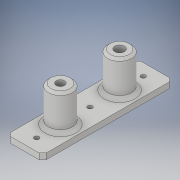
# Autodesk Inventor part: Part2
Saved by Autodesk Inventor 2019 (Build 230136000, 136)
## iProperties
Created: 2018-10-08
Part Number: Part2
Material: Generic
Document SubType Name: Modeling
Designer: Steven
Density: 1 g/cm^3
Appearance: Default
Author: Steven
## iProperties of the stored document Part2_3DPrint.ipt
Created: 2018-10-11
Part Number: Part2_3DPrint
Material: Generic
Document SubType Name: Modeling
Designer: Steven
Density: 1 g/cm^3
Appearance: Default
Author: Steven
Autodesk Inventor part; units mm, degrees
ref_plane "YZ Plane" through (0, 0, 0) normal (1, 0, 0) x (0, 1, 0)
ref_plane "XZ Plane" through (0, 0, 0) normal (0, 1, 0) x (-1, 0, 0)
ref_plane "XY Plane" through (0, 0, 0) normal (0, 0, 1) x (1, 0, 0)
sketch "Sketch1" plane through (0, 0, 0) normal (0, 1, 0) x (-1, 0, 0)
  line L0 (0, 0) -> (30, 0)
  line L1 (30, 0) -> (30, -110)
  line L2 (30, -110) -> (0, -110)
  line L3 (0, -110) -> (0, 0)
  dimension "d0" = 30
  dimension "d1" = 110
  constraints: 8 end point, 2 parallel, 1 horizontal, 1 perpendicular
  measures "d0" distance of L1.end L2.end
  measures "d1" distance of L0.end L1.end
extrude "Extrusion1" add sketch "Sketch1" along normal blind 5
sketch "Sketch2" plane through (0, 5, 0) normal (0, 1, 0) x (1, 0, 0)
  circle A0 centre (-10, 30) radius 3.5
  line L0 (0, 0) -> (0, 110) projected
  line L1 (-30, 0) -> (0, 0) projected
  circle A1 centre (-10, 30) radius 20
  line L2 (-30, 110) -> (-30, 0) projected
  circle A2 centre (-15, 10) radius 2
  line L3 (-30, 55) -> (0, 55) construction
  circle A3 centre (-10, 80) radius 3.5
  circle A4 centre (-10, 80) radius 20
  circle A5 centre (-15, 100) radius 2
  circle A6 centre (-15, 55) radius 2
  line L4 (-15, 0) -> (-15, 110) construction
  dimension "d4" = 7
  dimension "d5" = 10
  dimension "d6" = 30
  dimension "d7" = 4
  dimension "d9" = 10
  dimension "d10" = 4
  constraints: 7 centre point, 4 end point, 4 midpoint, 2 symmetric about line, 1 point on line, 1 tangent, 1 vertical, 3 other
  measures "d4" diameter of A0
  measures "d5" distance from line of L0 A0.centre
  measures "d6" distance from line of L1 A0.centre
  measures "d7" diameter of A2
  measures "d9" distance from line of L1 A2.centre
  measures "d10" diameter of A6
extrude "Extrusion2" cut sketch "Sketch2" against normal blind 5 contours A2 A1 | A1 A2 | A5 A4 | A4 A5 | A6
sketch "Sketch3" plane through (0, 5, 0) normal (0, 1, 0) x (1, 0, 0)
  line L0 (0, 110) -> (0, 0) construction
  line L1 (0, 55) -> (-30, 55) construction
  line L2 (-30, 0) -> (-30, 110) construction
  circle A0 centre (-15, 30) radius 3.5
  circle A1 centre (-15, 80) radius 4.1
  line L3 (-30, 0) -> (0, 0) projected
  line L4 (0, 110) -> (-30, 110) projected
  circle A2 centre (-15, 30) radius 10
  circle A3 centre (-15, 80) radius 10
  line L5 (-30, 110) -> (-30, 0) projected
  line L6 (-15, 0) -> (-15, 110) construction
  dimension "d13" = 7
  dimension "d14" = 8.2
  dimension "d16" = 30
  dimension "d17" = 30
  dimension "d22" = 20
  constraints: 4 centre point, 4 end point, 4 midpoint, 2 point on line, 1 equal radius
  measures "d13" diameter of A0
  measures "d14" diameter of A1
  measures "d16" distance from line of L3 A0.centre
  measures "d17" distance from line of L4 A1.centre
  measures "d22" diameter of A3
extrude "Extrusion3" add sketch "Sketch3" along normal blind 30
chamfer "Chamfer1" distance 3 angle 45 1 edges at (-25, 5, -30)
chamfer "Chamfer2" distance 3 angle 45 1 edges at (-25, 5, -80)
chamfer "Chamfer3" distance 3 angle 45 4 edges at (-30, 2.5, 0) (0, 2.5, 0) (0, 2.5, -110) (-30, 2.5, -110)
chamfer "Chamfer4" distance 2 angle 45 2 edges at (-25, 35, -80) (-25, 35, -30)
body "Solid1"
